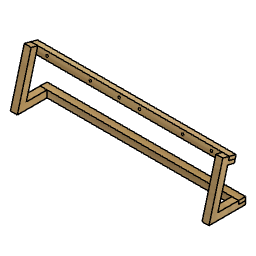
BTC ETH Ticker Stand v9 (Autodesk Fusion 360 design; units mm, degrees)
Autodesk Fusion 360 part; units mm, degrees
note: some values were not read from the file. Set by a fixed rule: which sketch regions a step uses.
sketch "Sketch1" plane through (0, 0, 0) normal (1, 0, 0) x (0, 1, 0)
  line L0 (0, 0) -> (23.9951, 89.551)
  line L1 (23.9951, 89.551) -> (35.5263, 86.4612)
  line L2 (35.5263, 86.4612) -> (15.5579, 11.938)
  line L3 (15.5579, 11.938) -> (51.562, 11.938)
  line L4 (63.5, 5.969) -> (63.5, 0)
  line L5 (63.5, 0) -> (0, 0)
  line L6 (45.5127, 77.6058) -> (43.9678, 71.8402)
  line L7 (43.9678, 71.8402) -> (32.4366, 74.93)
  line L8 (45.5127, 77.6058) -> (33.9814, 80.6956)
  line L9 (63.5, 5.969) -> (51.562, 5.969)
  line L10 (51.562, 5.969) -> (51.562, 11.938)
  dimension "d9" = 92.71
  dimension "d10" = 11.938
  dimension "d11" = 75
  dimension "d13" = 63.5
  dimension "d24" = 11.938
  dimension "d25" = 5.969
  dimension "d26" = 5.969
  dimension "d27" = 11.938
  dimension "d28" = 5.969
  dimension "d29" = 36.0041
  constraint coincident L0.start L5.end
  constraint perpendicular L0 L1
  constraint perpendicular L1 L2
  constraint horizontal L3
  constraint perpendicular L3 L4
  constraint perpendicular L4 L5
  constraint coincident L2 L7.end
  constraint perpendicular L2 L7
  constraint coincident L2 L8.end
  constraint perpendicular L2 L8
  constraint perpendicular L4 L9
  constraint perpendicular L3 L10
  measures "d9" distance of L0.start L0.end
  measures "d10" distance of L0.end L1.end
  measures "d11" angle of L2 L3
  measures "d13" distance of L4.end L0.start
  measures "d24" distance of L6.end L7.end
  measures "d25" distance of L6.end L6.start
  measures "d26" distance of L1 L8
  measures "d27" distance of L4.start L9.end
  measures "d28" distance of L4.end L4.start
  measures "d29" distance of L2.end L3.end
extrude "Extrude1" add sketch "Sketch1" along normal blind 11.938 makes body 1
sketch "Sketch3" plane through (0, 23.0624, -6.1796) normal (0, 0.965926, -0.258819) x (-1, 0, 0)
  line L0 (0, 80.772) -> (0, 86.741)
  line L1 (-11.938, 86.741) -> (-11.938, 80.772)
  line L2 (-11.938, 80.772) -> (0, 80.772)
  line L3 (0, 80.772) -> (-344.551, 80.772)
  line L4 (-344.551, 80.772) -> (-344.551, 92.71)
  line L5 (-344.551, 92.71) -> (0, 92.71)
  line L6 (0, 92.71) -> (0, 80.772)
  line L7 (0, 86.741) -> (-11.938, 86.741)
  dimension "d16" = 11.938
  dimension "d17" = 344.551
  constraint horizontal L3
  constraint vertical L4
  constraint horizontal L5
  constraint vertical L6
  constraint coincident L0.start L2.end
  measures "d16" distance of L0.start L5.end
  measures "d17" distance of L4.end L5.end
extrude "Extrude3" add sketch "Sketch3" against normal blind 11.938 separate body makes body 2
ref_plane "WorkPlane2" through (172.2755, 39.7471, 79.1507) normal (-1, 0, 0) x (0, -0.258819, -0.965926)
mirror "Mirror2" about plane through (172.2755, 39.7471, 79.1507) normal (-1, 0, 0) of bodies 1 makes body 3
sketch "Sketch4" plane through (0, 0, 0) normal (-1, 0, 0) x (0, -1, 0)
  line L0 (-43.9678, 71.8402) -> (-32.4366, 74.93)
  line L1 (-32.4366, 74.93) -> (-15.5579, 11.938)
  line L2 (-15.5579, 11.938) -> (-51.562, 11.938)
  line L3 (-51.562, 11.938) -> (-51.562, 5.969)
  line L4 (-51.562, 5.969) -> (-63.5, 5.969)
  line L5 (-63.5, 5.969) -> (-63.5, 0)
  line L6 (-63.5, 0) -> (0, 0)
  line L7 (0, 0) -> (-23.9951, 89.551)
  line L8 (-23.9951, 89.551) -> (-35.5263, 86.4612)
  line L9 (-35.5263, 86.4612) -> (-33.9814, 80.6956)
  line L10 (-33.9814, 80.6956) -> (-45.5127, 77.6058)
  line L11 (-45.5127, 77.6058) -> (-43.9678, 71.8402)
  line L12 (-63.5, 0) -> (-51.562, 0)
  line L13 (-51.562, 0) -> (-51.562, 11.938)
  line L14 (-51.562, 11.938) -> (-63.5, 11.938)
  line L15 (-63.5, 11.938) -> (-63.5, 0)
  constraint horizontal L12
  constraint vertical L13
  constraint horizontal L14
  constraint vertical L15
  constraint coincident L2.end L3.start
  constraint coincident L5.end L6.start
extrude "Extrude4" add sketch "Sketch4" against normal up to surface (344.551 mm away) separate body contours L3 L4 L13 L14 L15 | L4 L5 L6 L12 L13 L15 makes body 4
combine "Combine3" operation cut target body 2 tool bodies 1 3 keep tools
combine "Combine4" operation cut target body 4 tool bodies 1 3 keep tools
copy_body "Body->Comp9" bodies 1 removing the originals makes body 5 in component "Side1"
copy_body "Body->Comp10" bodies 2 removing the originals makes body 6 in component "TopStretcher"
copy_body "Body->Comp11" bodies 3 removing the originals makes body 7 in component "Side2"
copy_body "Body->Comp12" bodies 4 removing the originals makes body 8 in component "BottomStretcher"
sketch "Sketch5" plane through (0, 11.5312, -3.0898) normal (0, -0.965926, 0.258819) x (1, 0, 0)
  line L0 (344.551, 92.71) -> (0, 92.71)
  line L1 (0, 92.71) -> (0, 86.741)
  line L2 (0, 86.741) -> (11.938, 86.741)
  line L3 (11.938, 86.741) -> (11.938, 80.772)
  line L4 (11.938, 80.772) -> (332.613, 80.772)
  line L5 (332.613, 80.772) -> (332.613, 86.741)
  line L6 (332.613, 86.741) -> (344.551, 86.741)
  line L7 (344.551, 86.741) -> (344.551, 92.71)
  line L8 (11.938, 86.741) -> (332.613, 86.741) construction
  circle A0 centre (314.9346, 86.741) radius 1.905
  circle A1 centre (264.9474, 86.741) radius 1.905
  circle A2 centre (189.9412, 86.741) radius 1.905
  circle A3 centre (29.6164, 86.741) radius 1.905
  circle A4 centre (104.5972, 86.741) radius 1.905
  circle A5 centre (154.6098, 86.741) radius 1.905
  line L9 (11.938, 92.71) -> (11.938, 0)
  dimension "d32" = 3.81
  dimension "d33" = 3.81
  dimension "d34" = 3.81
  dimension "d35" = 17.6784
  dimension "d36" = 67.6656
  dimension "d37" = 142.6718
  dimension "d42" = 3.81
  dimension "d43" = 3.81
  dimension "d44" = 3.81
  dimension "d45" = 17.6784
  dimension "d46" = 92.6592
  dimension "d47" = 142.6718
  constraint coincident L2.end L3.start
  constraint coincident L5.end L6.start
  constraint coincident L8 A0.centre
  constraint coincident L8 A1.centre
  constraint coincident L8 A2.centre
  constraint coincident L8 A3.centre
  constraint coincident L8 A4.centre
  constraint coincident L8 A5.centre
  measures "d32" diameter of A0
  measures "d33" diameter of A1
  measures "d34" diameter of A2
  measures "d35" distance of L5 A0.centre
  measures "d36" distance of L5 A1.centre
  measures "d37" distance of L5 A2.centre
  measures "d42" diameter of A3
  measures "d43" diameter of A4
  measures "d44" diameter of A5
  measures "d45" distance of L3 A3.centre
  measures "d46" distance of L3 A4.centre
  measures "d47" distance of A5.centre L9
extrude "Extrude1'" cut sketch "Sketch5" against normal through all contours A0 | A1 | A2 | A3 | A4 | A5 bodies 6 in component "TopStretcher"
component "Side1" placed x (1, 0, 0) y (0, 1, 0) z (0, 0, 1) at (0, 0, 0)
component "TopStretcher" placed x (1, 0, 0) y (0, 1, 0) z (0, 0, 1) at (0, 0, 0)
component "Side2" placed x (1, 0, 0) y (0, 1, 0) z (0, 0, 1) at (0, 0, 0)
component "BottomStretcher" placed x (1, 0, 0) y (0, 1, 0) z (0, 0, 1) at (0, 0, 0)
equation "PlyThin = 0.47 in"
equation "d2 = PlyThin"
equation "d9 = PanelHeight + 0.5 in"
equation "d10 = PlyThin"
equation "d16 = PlyThin"
equation "d17 = PanelWidth"
equation "PanelWidth = 2 * 6 5/16\" + 2 * PlyThin"
equation "PanelHeight = 3.15 in"
equation "d20 = -PlyThin"
equation "d24 = PlyThin"
equation "d25 = PlyThin / 2"
equation "d26 = PlyThin / 2"
equation "d27 = PlyThin"
equation "d28 = PlyThin / 2"
